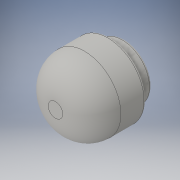
# Autodesk Inventor part: BottomStands
Saved by Autodesk Inventor 2016 (Build 200138000, 138)
## iProperties
Created: 2017-03-07
Part Number: BottomStands
Material: Generic
Document SubType Name: Modeling
Designer: peter
Density: 1 g/cm^3
Appearance: Default
Author: peter
Autodesk Inventor part; units mm, degrees
ref_plane "YZ Plane" through (0, 0, 0) normal (1, 0, 0) x (0, 1, 0)
ref_plane "XZ Plane" through (0, 0, 0) normal (0, 1, 0) x (-1, 0, 0)
ref_plane "XY Plane" through (0, 0, 0) normal (0, 0, 1) x (1, 0, 0)
sketch "Sketch1" plane through (0, 0, 0) normal (1, 0, 0) x (0, 1, 0)
  line L0 (0, 0) -> (0, 9.586) construction
  line L1 (0, 0) -> (4.3656, 0)
  line L2 (4.7625, 0.3969) -> (4.7625, 2.54)
  line L3 (4.7625, 2.54) -> (0, 2.54)
  line L4 (0, 2.54) -> (0, 0)
  line L5 (0, 2.54) -> (5.9531, 2.54)
  line L6 (6.35, 2.9369) -> (6.35, 6.985)
  line L7 (1.27, 12.065) -> (0, 12.065)
  line L8 (0, 12.065) -> (0, 2.54)
  arc A0 (4.3656, 0) -> (4.7625, 0.3969) centre (4.3656, 0.3969) ccw
  arc A1 (5.9531, 2.54) -> (6.35, 2.9369) centre (5.9531, 2.9369) ccw
  arc A2 (6.35, 6.985) -> (1.27, 12.065) centre (1.27, 6.985) ccw
  point P0 (4.7625, 0)
  point P1 (6.35, 12.065)
  point P2 (6.35, 2.54)
  point P3 (5.9531, 12.065)
  point P4 (6.35, 11.6681)
  dimension "d0" = 2.54
  dimension "d4" = 9.525
  dimension "d5" = 6.35
  dimension "d6" = 0.3969
  dimension "d7" = 0.3969
  dimension "d11" = 4.7625
  dimension "d14" = 5.08
  constraints: 18 end point, 8 point on line, 6 point on circle, 6 tangent, 4 parallel, 3 centre point, 2 horizontal, 2 perpendicular, 1 collinear, 1 vertical
  measures "d0" distance of point (4.763, 0) L2.end
  measures "d4" distance of point (6.35, 2.54) point (6.35, 12.065)
  measures "d5" distance between parallel lines of L0 L6
  measures "d6" radius of A0
  measures "d7" radius of A1
  measures "d11" distance between parallel lines of L0 L2
  measures "d14" radius of A2
revolve "Revolution1" add sketch "Sketch1" angle 360 about axis through (0, 0, 0) along (0, 0, 1)
body "Solid1"
